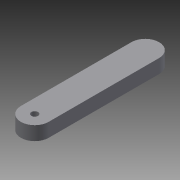
# Autodesk Inventor part: Fixture_Lever
Saved by Autodesk Inventor 2015 (Build 190159000, 159)
## iProperties
Created: 2014-12-16
Part Number: Fixture_Lever
Material: Generic
Document SubType Name: Modeling
Designer: amarschn
Density: 1 g/cm^3
Appearance: Default
Author: amarschn
Autodesk Inventor part; units mm, degrees
ref_plane "YZ Plane" through (0, 0, 0) normal (1, 0, 0) x (0, 1, 0)
ref_plane "XZ Plane" through (0, 0, 0) normal (0, 1, 0) x (-1, 0, 0)
ref_plane "XY Plane" through (0, 0, 0) normal (0, 0, 1) x (1, 0, 0)
sketch "Sketch1" plane through (0, 0, 0) normal (0, 1, 0) x (-1, 0, 0)
  line L0 (6.3636, -25.4) -> (6.3636, 25.4)
  line L1 (-6.3364, 25.2915) -> (-6.3364, -25.2915)
  line L2 (-6.3364, -25.2915) -> (6.3636, 25.4) construction
  line L3 (6.3636, -25.4) -> (-6.3364, 25.2915) construction
  arc A0 (6.3636, 25.4) -> (-6.3364, 25.2915) centre (0.0131, 25.4) ccw
  arc A1 (-6.3364, -25.2915) -> (6.3636, -25.4) centre (0.0131, -25.4) ccw
  circle A2 centre (0.0131, 25.4) radius 1.5434
  point P0 (0, 0)
  dimension "d0" = 50.8
  dimension "d1" = 12.7
  constraints: 8 end point, 4 point on circle, 3 centre point, 2 point on line, 2 tangent, 1 coincident, 1 parallel
  measures "d0" distance of A1.centre A0.centre
  measures "d1" distance between parallel lines of L1 L0
extrude "Extrusion1" add sketch "Sketch1" along normal blind 6.35
body "Solid1"
